Autodesk Inventor part; units mm, degrees
(part 2 of 2)
sketch "Sketch14" plane through (0, 5, 0) normal (0, 1, 0) x (1, 0, 0)
  line L0 (-61, 132) -> (-70, 132) construction
  line L1 (-70, 132) -> (-70, 8) construction
  line L2 (-70, 8) -> (-61, 8) construction
  line L3 (-61, 8) -> (-61, 10) construction
  line L4 (-61, 10) -> (-57, 10) construction
  line L5 (-57, 10) -> (-57, 8) construction
  line L6 (-57, 8) -> (-53, 8) construction
  line L7 (-53, 8) -> (-53, 4) construction
  line L8 (-53, 4) -> (-57, 4) construction
  line L9 (-57, 4) -> (-57, 2) construction
  line L10 (-57, 2) -> (-61, 2) construction
  line L11 (-61, 2) -> (-61, 4) construction
  line L12 (-61, 4) -> (-70, 4) construction
  line L13 (-70, 4) -> (-70, -36) construction
  line L14 (-70, -36) -> (-61, -36) construction
  line L15 (-61, -36) -> (-61, -34) construction
  line L16 (-61, -34) -> (-57, -34) construction
  line L17 (-57, -34) -> (-57, -36) construction
  line L18 (-57, -36) -> (-53, -36) construction
  line L19 (-53, -36) -> (-53, -40) construction
  line L20 (-53, -40) -> (-57, -40) construction
  line L21 (-57, -40) -> (-57, -42) construction
  line L22 (-57, -42) -> (-61, -42) construction
  line L23 (-61, -42) -> (-61, -40) construction
  line L24 (-61, -40) -> (-70, -40) construction
  line L25 (-70, -40) -> (-70, -60) construction
  line L26 (-70, -60) -> (230, -60) construction
  line L27 (230, -40) -> (230, -60) construction
  line L28 (230, -40) -> (221, -40) construction
  line L29 (221, -40) -> (221, -42) construction
  line L30 (221, -42) -> (217, -42) construction
  line L31 (217, -42) -> (217, -40) construction
  line L32 (217, -40) -> (213, -40) construction
  line L33 (213, -40) -> (213, -36) construction
  line L34 (213, -36) -> (217, -36) construction
  line L35 (217, -36) -> (217, -34) construction
  line L36 (217, -34) -> (221, -34) construction
  line L37 (221, -34) -> (221, -36) construction
  line L38 (221, -36) -> (230, -36) construction
  line L39 (230, 4) -> (230, -36) construction
  line L40 (230, 4) -> (221, 4) construction
  line L41 (221, 4) -> (221, 2) construction
  line L42 (221, 2) -> (217, 2) construction
  line L43 (217, 2) -> (217, 4) construction
  line L44 (217, 4) -> (213, 4) construction
  line L45 (213, 4) -> (213, 8) construction
  line L46 (213, 8) -> (217, 8) construction
  line L47 (217, 8) -> (217, 10) construction
  line L48 (217, 10) -> (221, 10) construction
  line L49 (221, 10) -> (221, 8) construction
  line L50 (221, 8) -> (230, 8) construction
  line L51 (230, 132) -> (230, 8) construction
  line L52 (230, 132) -> (221, 132) construction
  line L53 (221, 132) -> (221, 130) construction
  line L54 (221, 130) -> (217, 130) construction
  line L55 (217, 130) -> (217, 132) construction
  line L56 (217, 132) -> (213, 132) construction
  line L57 (213, 132) -> (213, 136) construction
  line L58 (213, 136) -> (217, 136) construction
  line L59 (217, 136) -> (217, 138) construction
  line L60 (217, 138) -> (221, 138) construction
  line L61 (221, 138) -> (221, 136) construction
  line L62 (221, 136) -> (230, 136) construction
  line L63 (230, 176) -> (230, 136) construction
  line L64 (230, 176) -> (221, 176) construction
  line L65 (221, 176) -> (221, 174) construction
  line L66 (221, 174) -> (217, 174) construction
  line L67 (217, 174) -> (217, 176) construction
  line L68 (217, 176) -> (213, 176) construction
  line L69 (213, 176) -> (213, 180) construction
  line L70 (213, 180) -> (217, 180) construction
  line L71 (217, 180) -> (217, 182) construction
  line L72 (217, 182) -> (221, 182) construction
  line L73 (221, 182) -> (221, 180) construction
  line L74 (221, 180) -> (230, 180) construction
  line L75 (230, 200) -> (230, 180) construction
  line L76 (230, 200) -> (-70, 200) construction
  line L77 (-70, 200) -> (-70, 180) construction
  line L78 (-70, 180) -> (-61, 180) construction
  line L79 (-61, 180) -> (-61, 182) construction
  line L80 (-61, 182) -> (-57, 182) construction
  line L81 (-57, 182) -> (-57, 180) construction
  line L82 (-57, 180) -> (-53, 180) construction
  line L83 (-53, 180) -> (-53, 176) construction
  line L84 (-53, 176) -> (-57, 176) construction
  line L85 (-57, 176) -> (-57, 174) construction
  line L86 (-57, 174) -> (-61, 174) construction
  line L87 (-61, 174) -> (-61, 176) construction
  line L88 (-61, 176) -> (-70, 176) construction
  line L89 (-70, 176) -> (-70, 136) construction
  line L90 (-70, 136) -> (-61, 136) construction
  line L91 (-61, 136) -> (-61, 138) construction
  line L92 (-61, 138) -> (-57, 138) construction
  line L93 (-57, 138) -> (-57, 136) construction
  line L94 (-57, 136) -> (-53, 136) construction
  line L95 (-53, 136) -> (-53, 132) construction
  line L96 (-53, 132) -> (-57, 132) construction
  line L97 (-57, 132) -> (-57, 130) construction
  line L98 (-57, 130) -> (-61, 130) construction
  line L99 (-61, 130) -> (-61, 132) construction
  line L100 (214, 35) -> (214, 30) construction
  line L101 (214, 30) -> (196, 30) construction
  line L102 (196, 30) -> (196, 35) construction
  line L103 (196, 35) -> (214, 35) construction
  circle A0 centre (190, 107.5) radius 2 construction
  circle A1 centre (220, 32.5) radius 2 construction
  circle A2 centre (190, 32.5) radius 2 construction
  circle A3 centre (220, 107.5) radius 2 construction
  line L104 (196, 110) -> (214, 110) construction
  line L105 (214, 110) -> (214, 105) construction
  line L106 (214, 105) -> (196, 105) construction
  line L107 (196, 105) -> (196, 110) construction
  circle A4 centre (-51, 27.5) radius 2 construction
  circle A5 centre (-51, 112.5) radius 2 construction
  circle A6 centre (-19, 112.5) radius 2 construction
  circle A7 centre (-19, 27.5) radius 2 construction
  circle A8 centre (177.5, -45) radius 2 construction
  circle A9 centre (2.5, 185) radius 2 construction
  circle A10 centre (177.5, 185) radius 2 construction
  circle A11 centre (2.5, -45) radius 2 construction
  line L108 (0, 5) -> (0, 25) construction
  line L109 (0, 25) -> (5, 25) construction
  line L110 (5, 25) -> (5, 5) construction
  line L111 (5, 5) -> (0, 5) construction
  circle A12 centre (2.5, -5) radius 2 construction
  line L112 (5, 135) -> (5, 115) construction
  line L113 (5, 115) -> (0, 115) construction
  line L114 (0, 115) -> (0, 135) construction
  line L115 (5, 135) -> (0, 135) construction
  circle A13 centre (2.5, 145) radius 2 construction
  line L116 (175, 155) -> (175, 175) construction
  line L117 (175, 175) -> (180, 175) construction
  line L118 (180, 175) -> (180, 155) construction
  line L119 (180, 155) -> (175, 155) construction
  circle A14 centre (177.5, 145) radius 2 construction
  line L120 (175, 5) -> (175, 25) construction
  line L121 (175, 25) -> (180, 25) construction
  line L122 (180, 25) -> (180, 5) construction
  line L123 (180, 5) -> (175, 5) construction
  circle A15 centre (177.5, -5) radius 2 construction
  line L124 (175, 135) -> (180, 135) construction
  line L125 (180, 135) -> (180, 115) construction
  line L126 (180, 115) -> (175, 115) construction
  line L127 (175, 115) -> (175, 135) construction
  line L128 (0, 155) -> (5, 155) construction
  line L129 (0, 155) -> (0, 175) construction
  line L130 (0, 175) -> (5, 175) construction
  line L131 (5, 175) -> (5, 155) construction
  line L132 (0, -15) -> (5, -15) construction
  line L133 (5, -15) -> (5, -35) construction
  line L134 (5, -35) -> (0, -35) construction
  line L135 (0, -35) -> (0, -15) construction
  line L136 (175, -15) -> (180, -15) construction
  line L137 (180, -15) -> (180, -35) construction
  line L138 (180, -35) -> (175, -35) construction
  line L139 (175, -35) -> (175, -15) construction
  line L140 (-45, 25) -> (-45, 30) construction
  line L141 (-45, 30) -> (-25, 30) construction
  line L142 (-25, 30) -> (-25, 25) construction
  line L143 (-25, 25) -> (-45, 25) construction
  line L144 (-45, 110) -> (-45, 115) construction
  line L145 (-45, 115) -> (-25, 115) construction
  line L146 (-25, 115) -> (-25, 110) construction
  line L147 (-25, 110) -> (-45, 110) construction
  line L148 (-70, 70) -> (230, 70) construction
  line L149 (-70, 176) -> (-70, 136) projected
  line L150 (-70, 166) -> (-73.5, 166)
  line L151 (-73.5, 166) -> (-73.5, 146)
  line L152 (-73.5, 146) -> (-70, 146)
  line L153 (-70, 146) -> (-70, 166)
  line L154 (-70, -6) -> (-73.5, -6)
  line L155 (-73.5, -6) -> (-73.5, -26)
  line L156 (-73.5, -26) -> (-70, -26)
  line L157 (-70, -26) -> (-70, -6)
  line L158 (-70, 132) -> (-70, 8) projected
  line L159 (-70, 100) -> (-73.5, 100)
  line L160 (-73.5, 100) -> (-73.5, 40)
  line L161 (-73.5, 40) -> (-70, 40)
  line L162 (-70, 40) -> (-70, 100)
  line L163 (230, 200) -> (-70, 200) construction
  line L164 (80, 200) -> (80, -60) construction
  line L165 (221, 132) -> (230, 132) construction
  line L166 (230, 132) -> (230, 8) construction
  line L167 (230, 8) -> (221, 8) construction
  line L168 (221, 8) -> (221, 10) construction
  line L169 (221, 10) -> (217, 10) construction
  line L170 (217, 10) -> (217, 8) construction
  line L171 (217, 8) -> (213, 8) construction
  line L172 (213, 8) -> (213, 4) construction
  line L173 (213, 4) -> (217, 4) construction
  line L174 (217, 4) -> (217, 2) construction
  line L175 (217, 2) -> (221, 2) construction
  line L176 (221, 2) -> (221, 4) construction
  line L177 (221, 4) -> (230, 4) construction
  line L178 (230, 4) -> (230, -36) construction
  line L179 (230, -36) -> (221, -36) construction
  line L180 (221, -36) -> (221, -34) construction
  line L181 (221, -34) -> (217, -34) construction
  line L182 (217, -34) -> (217, -36) construction
  line L183 (217, -36) -> (213, -36) construction
  line L184 (230, 136) -> (221, 136) construction
  line L185 (221, 136) -> (221, 138) construction
  line L186 (221, 138) -> (217, 138) construction
  line L187 (217, 138) -> (217, 136) construction
  line L188 (217, 136) -> (213, 136) construction
  line L189 (213, 136) -> (213, 132) construction
  line L190 (213, 132) -> (217, 132) construction
  line L191 (217, 132) -> (217, 130) construction
  line L192 (217, 130) -> (221, 130) construction
  line L193 (221, 130) -> (221, 132) construction
  line L194 (230, 166) -> (233.5, 166)
  line L195 (233.5, 166) -> (233.5, 146)
  line L196 (233.5, 146) -> (230, 146)
  line L197 (230, 146) -> (230, 166)
  line L198 (230, -6) -> (233.5, -6)
  line L199 (233.5, -6) -> (233.5, -26)
  line L200 (233.5, -26) -> (230, -26)
  line L201 (230, -26) -> (230, -6)
  line L202 (230, 132) -> (230, 8)
  line L203 (230, 100) -> (233.5, 100)
  line L204 (233.5, 100) -> (233.5, 40)
  line L205 (233.5, 40) -> (230, 40)
  line L206 (230, 40) -> (230, 100)
  point P0 (0, 0)
  dimension "d139" = 3.5
  dimension "d140" = 20
  dimension "d141" = 3.5
  dimension "d142" = 20
  dimension "d143" = 3.5
  dimension "d144" = 60
  dimension "d145" = 30
  dimension "d171" = 10
  dimension "d172" = 10
  constraints: 112 end point, 12 symmetric about line, 6 parallel, 5 point on line, 4 midpoint, 3 horizontal, 3 perpendicular
  measures "d139" distance of L152.end L151.end
  measures "d140" distance of L151.end L150.end
  measures "d141" distance of L156.end L155.end
  measures "d142" distance of L155.end L154.end
  measures "d143" distance of L161.end L160.end
  measures "d144" distance of L160.end L159.end
  measures "d145" distance between parallel lines of L148 L159
  measures "d171" distance between parallel lines of L154 L12
  measures "d172" distance between parallel lines of L150 L88
extrude "Extrusion15" add sketch "Sketch14" against normal blind 5
sketch "Sketch15" plane through (0, 5, 0) normal (0, 1, 0) x (1, 0, 0)
  line L0 (-61, 132) -> (-70, 132) construction
  line L1 (-70, 132) -> (-70, 100) construction
  line L2 (-70, 100) -> (-73.5, 100) construction
  line L3 (-73.5, 100) -> (-73.5, 40) construction
  line L4 (-73.5, 40) -> (-70, 40) construction
  line L5 (-70, 40) -> (-70, 8) construction
  line L6 (-70, 8) -> (-61, 8) construction
  line L7 (-61, 8) -> (-61, 10) construction
  line L8 (-61, 10) -> (-57, 10) construction
  line L9 (-57, 10) -> (-57, 8) construction
  line L10 (-57, 8) -> (-53, 8) construction
  line L11 (-53, 8) -> (-53, 4) construction
  line L12 (-53, 4) -> (-57, 4) construction
  line L13 (-57, 4) -> (-57, 2) construction
  line L14 (-57, 2) -> (-61, 2) construction
  line L15 (-61, 2) -> (-61, 4) construction
  line L16 (-61, 4) -> (-70, 4) construction
  line L17 (-70, 4) -> (-70, -6) construction
  line L18 (-70, -6) -> (-73.5, -6) construction
  line L19 (-73.5, -6) -> (-73.5, -26) construction
  line L20 (-73.5, -26) -> (-70, -26) construction
  line L21 (-70, -26) -> (-70, -36) construction
  line L22 (-70, -36) -> (-61, -36) construction
  line L23 (-61, -36) -> (-61, -34) construction
  line L24 (-61, -34) -> (-57, -34) construction
  line L25 (-57, -34) -> (-57, -36) construction
  line L26 (-57, -36) -> (-53, -36) construction
  line L27 (-53, -36) -> (-53, -40) construction
  line L28 (-53, -40) -> (-57, -40) construction
  line L29 (-57, -40) -> (-57, -42) construction
  line L30 (-57, -42) -> (-61, -42) construction
  line L31 (-61, -42) -> (-61, -40) construction
  line L32 (-61, -40) -> (-70, -40) construction
  line L33 (-70, -40) -> (-70, -60) construction
  line L34 (-70, -60) -> (230, -60) construction
  line L35 (230, -40) -> (230, -60) construction
  line L36 (230, -40) -> (221, -40) construction
  line L37 (221, -40) -> (221, -42) construction
  line L38 (221, -42) -> (217, -42) construction
  line L39 (217, -42) -> (217, -40) construction
  line L40 (217, -40) -> (213, -40) construction
  line L41 (213, -40) -> (213, -36) construction
  line L42 (213, -36) -> (217, -36) construction
  line L43 (217, -36) -> (217, -34) construction
  line L44 (217, -34) -> (221, -34) construction
  line L45 (221, -34) -> (221, -36) construction
  line L46 (221, -36) -> (230, -36) construction
  line L47 (230, -26) -> (230, -36) construction
  line L48 (233.5, -26) -> (230, -26) construction
  line L49 (233.5, -6) -> (233.5, -26) construction
  line L50 (230, -6) -> (233.5, -6) construction
  line L51 (230, 4) -> (230, -6) construction
  line L52 (230, 4) -> (221, 4) construction
  line L53 (221, 4) -> (221, 2) construction
  line L54 (221, 2) -> (217, 2) construction
  line L55 (217, 2) -> (217, 4) construction
  line L56 (217, 4) -> (213, 4) construction
  line L57 (213, 4) -> (213, 8) construction
  line L58 (213, 8) -> (217, 8) construction
  line L59 (217, 8) -> (217, 10) construction
  line L60 (217, 10) -> (221, 10) construction
  line L61 (221, 10) -> (221, 8) construction
  line L62 (221, 8) -> (230, 8) construction
  line L63 (230, 40) -> (230, 8) construction
  line L64 (230, 40) -> (233.5, 40) construction
  line L65 (233.5, 40) -> (233.5, 100) construction
  line L66 (233.5, 100) -> (230, 100) construction
  line L67 (230, 132) -> (230, 100) construction
  line L68 (230, 132) -> (221, 132) construction
  line L69 (221, 132) -> (221, 130) construction
  line L70 (221, 130) -> (217, 130) construction
  line L71 (217, 130) -> (217, 132) construction
  line L72 (217, 132) -> (213, 132) construction
  line L73 (213, 132) -> (213, 136) construction
  line L74 (213, 136) -> (217, 136) construction
  line L75 (217, 136) -> (217, 138) construction
  line L76 (217, 138) -> (221, 138) construction
  line L77 (221, 138) -> (221, 136) construction
  line L78 (221, 136) -> (230, 136) construction
  line L79 (230, 146) -> (230, 136) construction
  line L80 (230, 146) -> (233.5, 146) construction
  line L81 (233.5, 146) -> (233.5, 166) construction
  line L82 (233.5, 166) -> (230, 166) construction
  line L83 (230, 176) -> (230, 166) construction
  line L84 (230, 176) -> (221, 176) construction
  line L85 (221, 176) -> (221, 174) construction
  line L86 (221, 174) -> (217, 174) construction
  line L87 (217, 174) -> (217, 176) construction
  line L88 (217, 176) -> (213, 176) construction
  line L89 (213, 176) -> (213, 180) construction
  line L90 (213, 180) -> (217, 180) construction
  line L91 (217, 180) -> (217, 182) construction
  line L92 (217, 182) -> (221, 182) construction
  line L93 (221, 182) -> (221, 180) construction
  line L94 (221, 180) -> (230, 180) construction
  line L95 (230, 200) -> (230, 180) construction
  line L96 (230, 200) -> (-70, 200) construction
  line L97 (-70, 200) -> (-70, 180) construction
  line L98 (-70, 180) -> (-61, 180) construction
  line L99 (-61, 180) -> (-61, 182) construction
  line L100 (-61, 182) -> (-57, 182) construction
  line L101 (-57, 182) -> (-57, 180) construction
  line L102 (-57, 180) -> (-53, 180) construction
  line L103 (-53, 180) -> (-53, 176) construction
  line L104 (-53, 176) -> (-57, 176) construction
  line L105 (-57, 176) -> (-57, 174) construction
  line L106 (-57, 174) -> (-61, 174) construction
  line L107 (-61, 174) -> (-61, 176) construction
  line L108 (-61, 176) -> (-70, 176) construction
  line L109 (-70, 176) -> (-70, 166) construction
  line L110 (-70, 166) -> (-73.5, 166) construction
  line L111 (-73.5, 166) -> (-73.5, 146) construction
  line L112 (-73.5, 146) -> (-70, 146) construction
  line L113 (-70, 146) -> (-70, 136) construction
  line L114 (-70, 136) -> (-61, 136) construction
  line L115 (-61, 136) -> (-61, 138) construction
  line L116 (-61, 138) -> (-57, 138) construction
  line L117 (-57, 138) -> (-57, 136) construction
  line L118 (-57, 136) -> (-53, 136) construction
  line L119 (-53, 136) -> (-53, 132) construction
  line L120 (-53, 132) -> (-57, 132) construction
  line L121 (-57, 132) -> (-57, 130) construction
  line L122 (-57, 130) -> (-61, 130) construction
  line L123 (-61, 130) -> (-61, 132) construction
  line L124 (214, 35) -> (214, 30) construction
  line L125 (214, 30) -> (196, 30) construction
  line L126 (196, 30) -> (196, 35) construction
  line L127 (196, 35) -> (214, 35) construction
  circle A0 centre (190, 107.5) radius 2 construction
  circle A1 centre (220, 32.5) radius 2 construction
  circle A2 centre (190, 32.5) radius 2 construction
  circle A3 centre (220, 107.5) radius 2 construction
  line L128 (196, 110) -> (214, 110) construction
  line L129 (214, 110) -> (214, 105) construction
  line L130 (214, 105) -> (196, 105) construction
  line L131 (196, 105) -> (196, 110) construction
  circle A4 centre (-51, 27.5) radius 2 construction
  circle A5 centre (-51, 112.5) radius 2 construction
  circle A6 centre (-19, 112.5) radius 2 construction
  circle A7 centre (-19, 27.5) radius 2 construction
  circle A8 centre (177.5, -45) radius 2 construction
  circle A9 centre (2.5, 185) radius 2 construction
  circle A10 centre (177.5, 185) radius 2 construction
  circle A11 centre (2.5, -45) radius 2 construction
  line L132 (0, 5) -> (0, 25) construction
  line L133 (0, 25) -> (5, 25) construction
  line L134 (5, 25) -> (5, 5) construction
  line L135 (5, 5) -> (0, 5) construction
  circle A12 centre (2.5, -5) radius 2 construction
  line L136 (5, 135) -> (5, 115) construction
  line L137 (5, 115) -> (0, 115) construction
  line L138 (0, 115) -> (0, 135) construction
  line L139 (5, 135) -> (0, 135) construction
  circle A13 centre (2.5, 145) radius 2 construction
  line L140 (175, 155) -> (175, 175) construction
  line L141 (175, 175) -> (180, 175) construction
  line L142 (180, 175) -> (180, 155) construction
  line L143 (180, 155) -> (175, 155) construction
  circle A14 centre (177.5, 145) radius 2 construction
  line L144 (175, 5) -> (175, 25) construction
  line L145 (175, 25) -> (180, 25) construction
  line L146 (180, 25) -> (180, 5) construction
  line L147 (180, 5) -> (175, 5) construction
  circle A15 centre (177.5, -5) radius 2 construction
  line L148 (175, 135) -> (180, 135) construction
  line L149 (180, 135) -> (180, 115) construction
  line L150 (180, 115) -> (175, 115) construction
  line L151 (175, 115) -> (175, 135) construction
  line L152 (0, 155) -> (5, 155) construction
  line L153 (0, 155) -> (0, 175) construction
  line L154 (0, 175) -> (5, 175) construction
  line L155 (5, 175) -> (5, 155) construction
  line L156 (0, -15) -> (5, -15) construction
  line L157 (5, -15) -> (5, -35) construction
  line L158 (5, -35) -> (0, -35) construction
  line L159 (0, -35) -> (0, -15) construction
  line L160 (175, -15) -> (180, -15) construction
  line L161 (180, -15) -> (180, -35) construction
  line L162 (180, -35) -> (175, -35) construction
  line L163 (175, -35) -> (175, -15) construction
  line L164 (-45, 25) -> (-45, 30) construction
  line L165 (-45, 30) -> (-25, 30) construction
  line L166 (-25, 30) -> (-25, 25) construction
  line L167 (-25, 25) -> (-45, 25) construction
  line L168 (-45, 110) -> (-45, 115) construction
  line L169 (-45, 115) -> (-25, 115) construction
  line L170 (-25, 115) -> (-25, 110) construction
  line L171 (-25, 110) -> (-45, 110) construction
  line L172 (230, 200) -> (-70, 200) construction
  line L173 (-30, 200) -> (30, 200)
  line L174 (30, 200) -> (30, 203.5)
  line L175 (30, 203.5) -> (-30, 203.5)
  line L176 (-30, 203.5) -> (-30, 200)
  line L177 (130, 200) -> (190, 200)
  line L178 (190, 200) -> (190, 203.5)
  line L179 (190, 203.5) -> (130, 203.5)
  line L180 (130, 203.5) -> (130, 200)
  line L181 (80, 200) -> (80, -60) construction
  line L182 (-70, -60) -> (230, -60) construction
  line L183 (-73.5, 70) -> (233.5, 70) construction
  line L184 (-30, -60) -> (30, -60)
  line L185 (30, -60) -> (30, -63.5)
  line L186 (30, -63.5) -> (-30, -63.5)
  line L187 (-30, -63.5) -> (-30, -60)
  line L188 (130, -60) -> (190, -60)
  line L189 (190, -60) -> (190, -63.5)
  line L190 (190, -63.5) -> (130, -63.5)
  line L191 (130, -63.5) -> (130, -60)
  point P0 (0, 0)
  dimension "d148" = 60
  dimension "d149" = 3.5
  dimension "d150" = 60
  dimension "d151" = 3.5
  dimension "d152" = 40
  dimension "d153" = 40
  constraints: 36 end point, 8 symmetric about line, 4 midpoint, 4 parallel, 2 horizontal, 2 perpendicular, 2 point on line
  measures "d148" distance of L175.end L174.end
  measures "d149" distance of L174.end L173.end
  measures "d150" distance of L179.end L178.end
  measures "d151" distance of L178.end L177.end
  measures "d152" distance between parallel lines of L97 L176
  measures "d153" distance between parallel lines of L95 L178
extrude "Extrusion16" add sketch "Sketch15" against normal blind 5
sketch "Sketch16" plane through (0, 5, 0) normal (0, 1, 0) x (1, 0, 0)
  line L0 (-61, 132) -> (-70, 132) construction
  line L1 (-70, 132) -> (-70, 100) construction
  line L2 (-70, 100) -> (-73.5, 100) construction
  line L3 (-73.5, 100) -> (-73.5, 40) construction
  line L4 (-73.5, 40) -> (-70, 40) construction
  line L5 (-70, 40) -> (-70, 8) construction
  line L6 (-70, 8) -> (-61, 8) construction
  line L7 (-61, 8) -> (-61, 10) construction
  line L8 (-61, 10) -> (-57, 10) construction
  line L9 (-57, 10) -> (-57, 8) construction
  line L10 (-57, 8) -> (-53, 8) construction
  line L11 (-53, 8) -> (-53, 4) construction
  line L12 (-53, 4) -> (-57, 4) construction
  line L13 (-57, 4) -> (-57, 2) construction
  line L14 (-57, 2) -> (-61, 2) construction
  line L15 (-61, 2) -> (-61, 4) construction
  line L16 (-61, 4) -> (-70, 4) construction
  line L17 (-70, 4) -> (-70, -6) construction
  line L18 (-70, -6) -> (-73.5, -6) construction
  line L19 (-73.5, -6) -> (-73.5, -26) construction
  line L20 (-73.5, -26) -> (-70, -26) construction
  line L21 (-70, -26) -> (-70, -36) construction
  line L22 (-70, -36) -> (-61, -36) construction
  line L23 (-61, -36) -> (-61, -34) construction
  line L24 (-61, -34) -> (-57, -34) construction
  line L25 (-57, -34) -> (-57, -36) construction
  line L26 (-57, -36) -> (-53, -36) construction
  line L27 (-53, -36) -> (-53, -40) construction
  line L28 (-53, -40) -> (-57, -40) construction
  line L29 (-57, -40) -> (-57, -42) construction
  line L30 (-57, -42) -> (-61, -42) construction
  line L31 (-61, -42) -> (-61, -40) construction
  line L32 (-61, -40) -> (-70, -40) construction
  line L33 (-70, -40) -> (-70, -60) construction
  line L34 (-70, -60) -> (-30, -60) construction
  line L35 (-30, -60) -> (-30, -63.5) construction
  line L36 (-30, -63.5) -> (30, -63.5) construction
  line L37 (30, -63.5) -> (30, -60) construction
  line L38 (30, -60) -> (130, -60) construction
  line L39 (130, -63.5) -> (130, -60) construction
  line L40 (190, -63.5) -> (130, -63.5) construction
  line L41 (190, -60) -> (190, -63.5) construction
  line L42 (190, -60) -> (230, -60) construction
  line L43 (230, -40) -> (230, -60) construction
  line L44 (230, -40) -> (221, -40) construction
  line L45 (221, -40) -> (221, -42) construction
  line L46 (221, -42) -> (217, -42) construction
  line L47 (217, -42) -> (217, -40) construction
  line L48 (217, -40) -> (213, -40) construction
  line L49 (213, -40) -> (213, -36) construction
  line L50 (213, -36) -> (217, -36) construction
  line L51 (217, -36) -> (217, -34) construction
  line L52 (217, -34) -> (221, -34) construction
  line L53 (221, -34) -> (221, -36) construction
  line L54 (221, -36) -> (230, -36) construction
  line L55 (230, -26) -> (230, -36) construction
  line L56 (233.5, -26) -> (230, -26) construction
  line L57 (233.5, -6) -> (233.5, -26) construction
  line L58 (230, -6) -> (233.5, -6) construction
  line L59 (230, 4) -> (230, -6) construction
  line L60 (230, 4) -> (221, 4) construction
  line L61 (221, 4) -> (221, 2) construction
  line L62 (221, 2) -> (217, 2) construction
  line L63 (217, 2) -> (217, 4) construction
  line L64 (217, 4) -> (213, 4) construction
  line L65 (213, 4) -> (213, 8) construction
  line L66 (213, 8) -> (217, 8) construction
  line L67 (217, 8) -> (217, 10) construction
  line L68 (217, 10) -> (221, 10) construction
  line L69 (221, 10) -> (221, 8) construction
  line L70 (221, 8) -> (230, 8) construction
  line L71 (230, 40) -> (230, 8) construction
  line L72 (230, 40) -> (233.5, 40) construction
  line L73 (233.5, 40) -> (233.5, 100) construction
  line L74 (233.5, 100) -> (230, 100) construction
  line L75 (230, 132) -> (230, 100) construction
  line L76 (230, 132) -> (221, 132) construction
  line L77 (221, 132) -> (221, 130) construction
  line L78 (221, 130) -> (217, 130) construction
  line L79 (217, 130) -> (217, 132) construction
  line L80 (217, 132) -> (213, 132) construction
  line L81 (213, 132) -> (213, 136) construction
  line L82 (213, 136) -> (217, 136) construction
  line L83 (217, 136) -> (217, 138) construction
  line L84 (217, 138) -> (221, 138) construction
  line L85 (221, 138) -> (221, 136) construction
  line L86 (221, 136) -> (230, 136) construction
  line L87 (230, 146) -> (230, 136) construction
  line L88 (230, 146) -> (233.5, 146) construction
  line L89 (233.5, 146) -> (233.5, 166) construction
  line L90 (233.5, 166) -> (230, 166) construction
  line L91 (230, 176) -> (230, 166) construction
  line L92 (230, 176) -> (221, 176) construction
  line L93 (221, 176) -> (221, 174) construction
  line L94 (221, 174) -> (217, 174) construction
  line L95 (217, 174) -> (217, 176) construction
  line L96 (217, 176) -> (213, 176) construction
  line L97 (213, 176) -> (213, 180) construction
  line L98 (213, 180) -> (217, 180) construction
  line L99 (217, 180) -> (217, 182) construction
  line L100 (217, 182) -> (221, 182) construction
  line L101 (221, 182) -> (221, 180) construction
  line L102 (221, 180) -> (230, 180) construction
  line L103 (230, 200) -> (230, 180) construction
  line L104 (230, 200) -> (190, 200) construction
  line L105 (190, 200) -> (190, 203.5) construction
  line L106 (190, 203.5) -> (130, 203.5) construction
  line L107 (130, 203.5) -> (130, 200) construction
  line L108 (130, 200) -> (30, 200) construction
  line L109 (30, 200) -> (30, 203.5) construction
  line L110 (30, 203.5) -> (-30, 203.5) construction
  line L111 (-30, 203.5) -> (-30, 200) construction
  line L112 (-30, 200) -> (-70, 200) construction
  line L113 (-70, 200) -> (-70, 180) construction
  line L114 (-70, 180) -> (-61, 180) construction
  line L115 (-61, 180) -> (-61, 182) construction
  line L116 (-61, 182) -> (-57, 182) construction
  line L117 (-57, 182) -> (-57, 180) construction
  line L118 (-57, 180) -> (-53, 180) construction
  line L119 (-53, 180) -> (-53, 176) construction
  line L120 (-53, 176) -> (-57, 176) construction
  line L121 (-57, 176) -> (-57, 174) construction
  line L122 (-57, 174) -> (-61, 174) construction
  line L123 (-61, 174) -> (-61, 176) construction
  line L124 (-61, 176) -> (-70, 176) construction
  line L125 (-70, 176) -> (-70, 166) construction
  line L126 (-70, 166) -> (-73.5, 166) construction
  line L127 (-73.5, 166) -> (-73.5, 146) construction
  line L128 (-73.5, 146) -> (-70, 146) construction
  line L129 (-70, 146) -> (-70, 136) construction
  line L130 (-70, 136) -> (-61, 136) construction
  line L131 (-61, 136) -> (-61, 138) construction
  line L132 (-61, 138) -> (-57, 138) construction
  line L133 (-57, 138) -> (-57, 136) construction
  line L134 (-57, 136) -> (-53, 136) construction
  line L135 (-53, 136) -> (-53, 132) construction
  line L136 (-53, 132) -> (-57, 132) construction
  line L137 (-57, 132) -> (-57, 130) construction
  line L138 (-57, 130) -> (-61, 130) construction
  line L139 (-61, 130) -> (-61, 132) construction
  line L140 (214, 35) -> (214, 30) construction
  line L141 (214, 30) -> (196, 30) construction
  line L142 (196, 30) -> (196, 35) construction
  line L143 (196, 35) -> (214, 35) construction
  circle A0 centre (190, 107.5) radius 2 construction
  circle A1 centre (220, 32.5) radius 2 construction
  circle A2 centre (190, 32.5) radius 2 construction
  circle A3 centre (220, 107.5) radius 2 construction
  line L144 (196, 110) -> (214, 110) construction
  line L145 (214, 110) -> (214, 105) construction
  line L146 (214, 105) -> (196, 105) construction
  line L147 (196, 105) -> (196, 110) construction
  circle A4 centre (-51, 27.5) radius 2 construction
  circle A5 centre (-51, 112.5) radius 2 construction
  circle A6 centre (-19, 112.5) radius 2 construction
  circle A7 centre (-19, 27.5) radius 2 construction
  circle A8 centre (177.5, -45) radius 2 construction
  circle A9 centre (2.5, 185) radius 2 construction
  circle A10 centre (177.5, 185) radius 2 construction
  circle A11 centre (2.5, -45) radius 2 construction
  line L148 (0, 5) -> (0, 25) construction
  line L149 (0, 25) -> (5, 25) construction
  line L150 (5, 25) -> (5, 5) construction
  line L151 (5, 5) -> (0, 5) construction
  circle A12 centre (2.5, -5) radius 2 construction
  line L152 (5, 135) -> (5, 115) construction
  line L153 (5, 115) -> (0, 115) construction
  line L154 (0, 115) -> (0, 135) construction
  line L155 (5, 135) -> (0, 135) construction
  circle A13 centre (2.5, 145) radius 2 construction
  line L156 (175, 155) -> (175, 175) construction
  line L157 (175, 175) -> (180, 175) construction
  line L158 (180, 175) -> (180, 155) construction
  line L159 (180, 155) -> (175, 155) construction
  circle A14 centre (177.5, 145) radius 2 construction
  line L160 (175, 5) -> (175, 25) construction
  line L161 (175, 25) -> (180, 25) construction
  line L162 (180, 25) -> (180, 5) construction
  line L163 (180, 5) -> (175, 5) construction
  circle A15 centre (177.5, -5) radius 2 construction
  line L164 (175, 135) -> (180, 135) construction
  line L165 (180, 135) -> (180, 115) construction
  line L166 (180, 115) -> (175, 115) construction
  line L167 (175, 115) -> (175, 135) construction
  line L168 (0, 155) -> (5, 155) construction
  line L169 (0, 155) -> (0, 175) construction
  line L170 (0, 175) -> (5, 175) construction
  line L171 (5, 175) -> (5, 155) construction
  line L172 (0, -15) -> (5, -15) construction
  line L173 (5, -15) -> (5, -35) construction
  line L174 (5, -35) -> (0, -35) construction
  line L175 (0, -35) -> (0, -15) construction
  line L176 (175, -15) -> (180, -15) construction
  line L177 (180, -15) -> (180, -35) construction
  line L178 (180, -35) -> (175, -35) construction
  line L179 (175, -35) -> (175, -15) construction
  line L180 (-45, 25) -> (-45, 30) construction
  line L181 (-45, 30) -> (-25, 30) construction
  line L182 (-25, 30) -> (-25, 25) construction
  line L183 (-25, 25) -> (-45, 25) construction
  line L184 (-45, 110) -> (-45, 115) construction
  line L185 (-45, 115) -> (-25, 115) construction
  line L186 (-25, 115) -> (-25, 110) construction
  line L187 (-25, 110) -> (-45, 110) construction
  line L188 (0, 25) -> (0, 5) construction
  line L189 (0, 115) -> (0, 25) construction
  line L190 (0, 100) -> (5, 100)
  line L191 (5, 100) -> (5, 40)
  line L192 (5, 40) -> (0, 40)
  line L193 (0, 40) -> (0, 100)
  point P0 (0, 0)
  dimension "d156" = 5
  dimension "d157" = 60
  dimension "d158" = 15
  constraints: 10 end point, 2 parallel, 1 collinear, 1 horizontal, 1 perpendicular, 1 point on line
  measures "d156" distance of L191.end L192.end
  measures "d157" distance of L190.end L191.end
  measures "d158" distance between parallel lines of L153 L190
extrude "Extrusion17" cut sketch "Sketch16" against normal blind 5
sketch "Sketch18" plane through (0, 5, 0) normal (0, 1, 0) x (1, 0, 0)
  line L0 (0, 40) -> (0, 100) construction
  line L1 (0, 100) -> (5, 100) construction
  line L2 (5, 100) -> (5, 40) construction
  line L3 (5, 40) -> (0, 40) construction
  line L4 (-61, 132) -> (-70, 132) construction
  line L5 (-70, 132) -> (-70, 100) construction
  line L6 (-70, 100) -> (-73.5, 100) construction
  line L7 (-73.5, 100) -> (-73.5, 40) construction
  line L8 (-73.5, 40) -> (-70, 40) construction
  line L9 (-70, 40) -> (-70, 8) construction
  line L10 (-70, 8) -> (-61, 8) construction
  line L11 (-61, 8) -> (-61, 10) construction
  line L12 (-61, 10) -> (-57, 10) construction
  line L13 (-57, 10) -> (-57, 8) construction
  line L14 (-57, 8) -> (-53, 8) construction
  line L15 (-53, 8) -> (-53, 4) construction
  line L16 (-53, 4) -> (-57, 4) construction
  line L17 (-57, 4) -> (-57, 2) construction
  line L18 (-57, 2) -> (-61, 2) construction
  line L19 (-61, 2) -> (-61, 4) construction
  line L20 (-61, 4) -> (-70, 4) construction
  line L21 (-70, 4) -> (-70, -6) construction
  line L22 (-70, -6) -> (-73.5, -6) construction
  line L23 (-73.5, -6) -> (-73.5, -26) construction
  line L24 (-73.5, -26) -> (-70, -26) construction
  line L25 (-70, -26) -> (-70, -36) construction
  line L26 (-70, -36) -> (-61, -36) construction
  line L27 (-61, -36) -> (-61, -34) construction
  line L28 (-61, -34) -> (-57, -34) construction
  line L29 (-57, -34) -> (-57, -36) construction
  line L30 (-57, -36) -> (-53, -36) construction
  line L31 (-53, -36) -> (-53, -40) construction
  line L32 (-53, -40) -> (-57, -40) construction
  line L33 (-57, -40) -> (-57, -42) construction
  line L34 (-57, -42) -> (-61, -42) construction
  line L35 (-61, -42) -> (-61, -40) construction
  line L36 (-61, -40) -> (-70, -40) construction
  line L37 (-70, -40) -> (-70, -60) construction
  line L38 (-70, -60) -> (-30, -60) construction
  line L39 (-30, -60) -> (-30, -63.5) construction
  line L40 (-30, -63.5) -> (30, -63.5) construction
  line L41 (30, -63.5) -> (30, -60) construction
  line L42 (30, -60) -> (130, -60) construction
  line L43 (130, -63.5) -> (130, -60) construction
  line L44 (190, -63.5) -> (130, -63.5) construction
  line L45 (190, -60) -> (190, -63.5) construction
  line L46 (190, -60) -> (230, -60) construction
  line L47 (230, -40) -> (230, -60) construction
  line L48 (230, -40) -> (221, -40) construction
  line L49 (221, -40) -> (221, -42) construction
  line L50 (221, -42) -> (217, -42) construction
  line L51 (217, -42) -> (217, -40) construction
  line L52 (217, -40) -> (213, -40) construction
  line L53 (213, -40) -> (213, -36) construction
  line L54 (213, -36) -> (217, -36) construction
  line L55 (217, -36) -> (217, -34) construction
  line L56 (217, -34) -> (221, -34) construction
  line L57 (221, -34) -> (221, -36) construction
  line L58 (221, -36) -> (230, -36) construction
  line L59 (230, -26) -> (230, -36) construction
  line L60 (233.5, -26) -> (230, -26) construction
  line L61 (233.5, -6) -> (233.5, -26) construction
  line L62 (230, -6) -> (233.5, -6) construction
  line L63 (230, 4) -> (230, -6) construction
  line L64 (230, 4) -> (221, 4) construction
  line L65 (221, 4) -> (221, 2) construction
  line L66 (221, 2) -> (217, 2) construction
  line L67 (217, 2) -> (217, 4) construction
  line L68 (217, 4) -> (213, 4) construction
  line L69 (213, 4) -> (213, 8) construction
  line L70 (213, 8) -> (217, 8) construction
  line L71 (217, 8) -> (217, 10) construction
  line L72 (217, 10) -> (221, 10) construction
  line L73 (221, 10) -> (221, 8) construction
  line L74 (221, 8) -> (230, 8) construction
  line L75 (230, 40) -> (230, 8) construction
  line L76 (230, 40) -> (233.5, 40) construction
  line L77 (233.5, 40) -> (233.5, 100) construction
  line L78 (233.5, 100) -> (230, 100) construction
  line L79 (230, 132) -> (230, 100) construction
  line L80 (230, 132) -> (221, 132) construction
  line L81 (221, 132) -> (221, 130) construction
  line L82 (221, 130) -> (217, 130) construction
  line L83 (217, 130) -> (217, 132) construction
  line L84 (217, 132) -> (213, 132) construction
  line L85 (213, 132) -> (213, 136) construction
  line L86 (213, 136) -> (217, 136) construction
  line L87 (217, 136) -> (217, 138) construction
  line L88 (217, 138) -> (221, 138) construction
  line L89 (221, 138) -> (221, 136) construction
  line L90 (221, 136) -> (230, 136) construction
  line L91 (230, 146) -> (230, 136) construction
  line L92 (230, 146) -> (233.5, 146) construction
  line L93 (233.5, 146) -> (233.5, 166) construction
  line L94 (233.5, 166) -> (230, 166) construction
  line L95 (230, 176) -> (230, 166) construction
  line L96 (230, 176) -> (221, 176) construction
  line L97 (221, 176) -> (221, 174) construction
  line L98 (221, 174) -> (217, 174) construction
  line L99 (217, 174) -> (217, 176) construction
  line L100 (217, 176) -> (213, 176) construction
  line L101 (213, 176) -> (213, 180) construction
  line L102 (213, 180) -> (217, 180) construction
  line L103 (217, 180) -> (217, 182) construction
  line L104 (217, 182) -> (221, 182) construction
  line L105 (221, 182) -> (221, 180) construction
  line L106 (221, 180) -> (230, 180) construction
  line L107 (230, 200) -> (230, 180) construction
  line L108 (230, 200) -> (190, 200) construction
  line L109 (190, 200) -> (190, 203.5) construction
  line L110 (190, 203.5) -> (130, 203.5) construction
  line L111 (130, 203.5) -> (130, 200) construction
  line L112 (130, 200) -> (30, 200) construction
  line L113 (30, 200) -> (30, 203.5) construction
  line L114 (30, 203.5) -> (-30, 203.5) construction
  line L115 (-30, 203.5) -> (-30, 200) construction
  line L116 (-30, 200) -> (-70, 200) construction
  line L117 (-70, 200) -> (-70, 180) construction
  line L118 (-70, 180) -> (-61, 180) construction
  line L119 (-61, 180) -> (-61, 182) construction
  line L120 (-61, 182) -> (-57, 182) construction
  line L121 (-57, 182) -> (-57, 180) construction
  line L122 (-57, 180) -> (-53, 180) construction
  line L123 (-53, 180) -> (-53, 176) construction
  line L124 (-53, 176) -> (-57, 176) construction
  line L125 (-57, 176) -> (-57, 174) construction
  line L126 (-57, 174) -> (-61, 174) construction
  line L127 (-61, 174) -> (-61, 176) construction
  line L128 (-61, 176) -> (-70, 176) construction
  line L129 (-70, 176) -> (-70, 166) construction
  line L130 (-70, 166) -> (-73.5, 166) construction
  line L131 (-73.5, 166) -> (-73.5, 146) construction
  line L132 (-73.5, 146) -> (-70, 146) construction
  line L133 (-70, 146) -> (-70, 136) construction
  line L134 (-70, 136) -> (-61, 136) construction
  line L135 (-61, 136) -> (-61, 138) construction
  line L136 (-61, 138) -> (-57, 138) construction
  line L137 (-57, 138) -> (-57, 136) construction
  line L138 (-57, 136) -> (-53, 136) construction
  line L139 (-53, 136) -> (-53, 132) construction
  line L140 (-53, 132) -> (-57, 132) construction
  line L141 (-57, 132) -> (-57, 130) construction
  line L142 (-57, 130) -> (-61, 130) construction
  line L143 (-61, 130) -> (-61, 132) construction
  line L144 (214, 35) -> (214, 30) construction
  line L145 (214, 30) -> (196, 30) construction
  line L146 (196, 30) -> (196, 35) construction
  line L147 (196, 35) -> (214, 35) construction
  circle A0 centre (190, 107.5) radius 2 construction
  circle A1 centre (220, 32.5) radius 2 construction
  circle A2 centre (190, 32.5) radius 2 construction
  circle A3 centre (220, 107.5) radius 2 construction
  line L148 (196, 110) -> (214, 110) construction
  line L149 (214, 110) -> (214, 105) construction
  line L150 (214, 105) -> (196, 105) construction
  line L151 (196, 105) -> (196, 110) construction
  circle A4 centre (-51, 27.5) radius 2 construction
  circle A5 centre (-51, 112.5) radius 2 construction
  circle A6 centre (-19, 112.5) radius 2 construction
  circle A7 centre (-19, 27.5) radius 2 construction
  circle A8 centre (177.5, -45) radius 2 construction
  circle A9 centre (2.5, 185) radius 2 construction
  circle A10 centre (177.5, 185) radius 2 construction
  circle A11 centre (2.5, -45) radius 2 construction
  line L152 (0, 5) -> (0, 25) construction
  line L153 (0, 25) -> (5, 25) construction
  line L154 (5, 25) -> (5, 5) construction
  line L155 (5, 5) -> (0, 5) construction
  circle A12 centre (2.5, -5) radius 2 construction
  line L156 (5, 135) -> (5, 115) construction
  line L157 (5, 115) -> (0, 115) construction
  line L158 (0, 115) -> (0, 135) construction
  line L159 (5, 135) -> (0, 135) construction
  circle A13 centre (2.5, 145) radius 2 construction
  line L160 (175, 155) -> (175, 175) construction
  line L161 (175, 175) -> (180, 175) construction
  line L162 (180, 175) -> (180, 155) construction
  line L163 (180, 155) -> (175, 155) construction
  circle A14 centre (177.5, 145) radius 2 construction
  line L164 (175, 5) -> (175, 25) construction
  line L165 (175, 25) -> (180, 25) construction
  line L166 (180, 25) -> (180, 5) construction
  line L167 (180, 5) -> (175, 5) construction
  circle A15 centre (177.5, -5) radius 2 construction
  line L168 (175, 135) -> (180, 135) construction
  line L169 (180, 135) -> (180, 115) construction
  line L170 (180, 115) -> (175, 115) construction
  line L171 (175, 115) -> (175, 135) construction
  line L172 (0, 155) -> (5, 155) construction
  line L173 (0, 155) -> (0, 175) construction
  line L174 (0, 175) -> (5, 175) construction
  line L175 (5, 175) -> (5, 155) construction
  line L176 (0, -15) -> (5, -15) construction
  line L177 (5, -15) -> (5, -35) construction
  line L178 (5, -35) -> (0, -35) construction
  line L179 (0, -35) -> (0, -15) construction
  line L180 (175, -15) -> (180, -15) construction
  line L181 (180, -15) -> (180, -35) construction
  line L182 (180, -35) -> (175, -35) construction
  line L183 (175, -35) -> (175, -15) construction
  line L184 (-45, 25) -> (-45, 30) construction
  line L185 (-45, 30) -> (-25, 30) construction
  line L186 (-25, 30) -> (-25, 25) construction
  line L187 (-25, 25) -> (-45, 25) construction
  line L188 (-45, 110) -> (-45, 115) construction
  line L189 (-45, 115) -> (-25, 115) construction
  line L190 (-25, 115) -> (-25, 110) construction
  line L191 (-25, 110) -> (-45, 110) construction
  line L192 (130, 200) -> (30, 200) construction
  line L193 (80, 200) -> (80, -60) construction
  line L194 (130, -60) -> (30, -60) construction
  line L195 (-73.5, 70) -> (233.5, 70) construction
  line L196 (40, 20) -> (36.5, 20)
  line L197 (36.5, 20) -> (36.5, 120)
  line L198 (36.5, 120) -> (40, 120)
  line L199 (40, 120) -> (40, 20)
  line L200 (78.25, 20) -> (81.75, 20)
  line L201 (81.75, 20) -> (81.75, 120)
  line L202 (81.75, 120) -> (78.25, 120)
  line L203 (78.25, 120) -> (78.25, 20)
  line L204 (123.5, 20) -> (120, 20)
  line L205 (120, 20) -> (120, 120)
  line L206 (120, 120) -> (123.5, 120)
  line L207 (123.5, 120) -> (123.5, 20)
  line L208 (123.5, 20) -> (120, 120) construction
  line L209 (120, 20) -> (123.5, 120) construction
  point P0 (0, 0)
  point P1 (44.3813, 70)
  point P2 (80, 70)
  point P3 (121.75, 70)
  dimension "d185" = 3.5
  dimension "d186" = 100
  dimension "d187" = 40
  dimension "d188" = 3.5
  dimension "d189" = 100
  dimension "d190" = 3.5
  dimension "d191" = 100
  dimension "d192" = 40
  constraints: 32 end point, 7 midpoint, 6 parallel, 3 horizontal, 3 perpendicular, 2 point on line
  measures "d185" distance of L197.end L198.end
  measures "d186" distance of L196.end L197.end
  measures "d187" distance between parallel lines of L193 L199
  measures "d188" distance of L202.end L201.end
  measures "d189" distance of L201.end L200.end
  measures "d190" distance of L205.end L206.end
  measures "d191" distance of L204.end L205.end
  measures "d192" distance between parallel lines of L193 L205
extrude "Extrusion19" cut sketch "Sketch18" against normal blind 5
body "Solid2"
